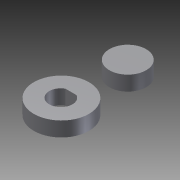
# Autodesk Inventor part: InputGear
Saved by Autodesk Inventor 2012 (Build 160160000, 160)
## iProperties
Created: 2011-10-22
Part Number: InputGear
Material: Default
Document SubType Name: Modeling
Designer: KuttaA
Density: 1 g/cm^3
Author: KuttaA
Autodesk Inventor part; units mm, degrees
ref_plane "YZ Plane" through (0, 0, 0) normal (1, 0, 0) x (0, 1, 0)
ref_plane "XZ Plane" through (0, 0, 0) normal (0, 1, 0) x (-1, 0, 0)
ref_plane "XY Plane" through (0, 0, 0) normal (0, 0, 1) x (1, 0, 0)
sketch "Sketch1" plane through (0, 0, 0) normal (0, 0, 1) x (1, 0, 0)
  line L0 (-1.7313, 2.45) -> (1.7313, 2.45) projected
  circle A0 centre (0, 0) radius 3 construction
  line L1 (-1.5362, 2.75) -> (1.5362, 2.75)
  arc A1 (-1.5362, 2.75) -> (1.5362, 2.75) centre (0, 0) ccw
  circle A2 centre (0.1509, 0) radius 7.5
  circle A3 centre (0.1509, 18.0718) radius 5
  dimension "d0" = 0.3
  dimension "d1" = 6
  dimension "d2" = 6.3
  dimension "d3" = 15
  dimension "d4" = 10
  constraints: 3 centre point, 3 coincident, 2 end point, 2 point on circle, 1 parallel
  measures "d0" distance between parallel lines of L1 L0
  measures "d1" diameter of A0
  measures "d2" diameter of A1
  measures "d3" diameter of A2
  measures "d4" diameter of A3
extrude "Extrusion1" add sketch "Sketch1" against normal blind 4
body "Solid1"
